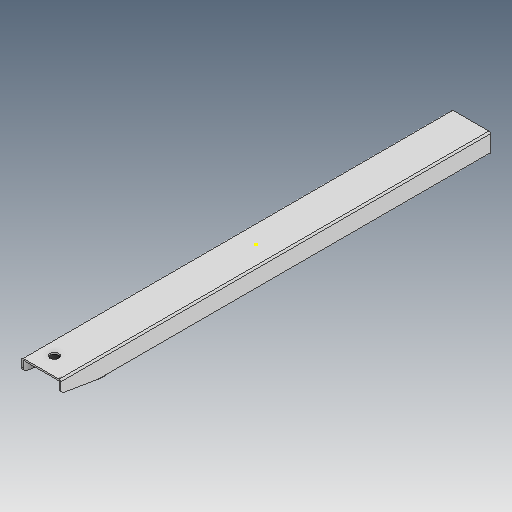
# Autodesk Inventor part: MC02-1
Saved by Autodesk Inventor 2020 (Build 240168000, 168)
## iProperties
Created: 2020-02-24
Part Number: MC02-1
Material: Generic
Document SubType Name: Modeling
Designer: Juan Carlos Botero
Density: 1 g/cm^3
Appearance: Default
Mass: 1184.23 g
Surface Area: 5972.04 cm^2
Volume: 1184.23 cm^3
Author: Juan Carlos Botero
Title: PERFIL SOPORTE BANDA (L)
Autodesk Inventor part; units mm, degrees
ref_plane "YZ Plane" through (0, 0, 0) normal (1, 0, 0) x (0, 1, 0)
ref_plane "XZ Plane" through (0, 0, 0) normal (0, 1, 0) x (-1, 0, 0)
ref_plane "XY Plane" through (0, 0, 0) normal (0, 0, 1) x (1, 0, 0)
sketch "Sketch1" plane through (0, 0, 0) normal (0, 0, 1) x (1, 0, 0)
  line L0 (-50, 25) -> (50, 25)
  line L1 (50, 25) -> (50, -25)
  line L2 (50, -25) -> (-50, -25)
  line L3 (-50, -25) -> (-50, 25)
  line L4 (-50, 25) -> (50, -25) construction
  line L5 (50, 25) -> (-50, -25) construction
  point P0 (0, 0)
  dimension "d0" = 100
  dimension "d1" = 50
  constraints: 12 end point, 2 midpoint, 2 parallel, 1 horizontal, 1 perpendicular
  measures "d0" distance of L1.end L2.end
  measures "d1" distance of L0.end L1.end
extrude "Extrusion1" add sketch "Sketch1" along normal mid plane 1100
fillet "Fillet1" radius 4 4 edges at (50, -25, 0) (50, 25, 0) (-50, -25, 0) (-50, 25, 0)
shell "Shell1" thickness 4 removed faces 2 at (-15.3333, -8.3333, 550) at (-15.3333, -8.3333, -550)
sketch "Sketch2" plane through (-46, 25, 550) normal (0, 1, 0) x (1, 0, 0)
  circle A0 centre (34.3509, 45.5772) radius 11.25 projected
  point P0 (46, 550)
extrude "Extrusion2" cut sketch "Sketch2" against normal through all
sketch "Sketch3" plane through (50, -21, 550) normal (1, 0, 0) x (0, 0, -1)
  line L0 (0, -4) -> (1100, -4) projected
  line L1 (0, 42) -> (0, 0) projected
  line L2 (0, 16) -> (120, -4)
  line L3 (0, -11.4428) -> (0, 16)
  line L4 (120, -4) -> (120, -11.4428)
  line L5 (120, -11.4428) -> (0, -11.4428)
  point P0 (550, 21)
  dimension "d8" = 120
  dimension "d9" = 20
  constraints: 8 end point, 3 point on line, 1 coincident, 1 horizontal, 1 vertical, 1 vertical alignment
  measures "d8" distance between parallel lines of L3 L4
  measures "d9" distance from line of point (0, 16) L0
extrude "Extrusion3" cut sketch "Sketch3" against normal blind 1100
fillet "Fillet2" radius 10 2 edges at (48, -5, 550) (-48, -5, 550)
sketch "Sketch4" plane through (-46, 25, 550) normal (0, 1, 0) x (1, 0, 0)
  line L0 (90.5966, 11.6068) -> (90.5966, 2.7213) construction
  line L1 (90.5966, 2.7213) -> (86.2672, 2.7213) construction
  line L2 (86.2672, 2.7213) -> (86.2672, 11.6068) construction
  line L3 (86.2672, 11.6068) -> (90.5966, 11.6068) construction
  point P0 (46, 550)
  constraints: 2 other
body "Solid1"
